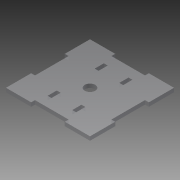
# Autodesk Inventor part: inside_box_top_bot
Saved by Autodesk Inventor 2013 (Build 170138000, 138)
## iProperties
Created: 2014-05-23
Part Number: inside_box_top_bot
Material: Polycarbonate, Clear
Document SubType Name: Modeling
Designer: balogh
Density: 0.894 g/cm^3
Mass: 9.34464 g
Surface Area: 83.2097 cm^2
Volume: 10.4526 cm^3
Author: balogh
Autodesk Inventor part; units mm, degrees
ref_plane "YZ Plane" through (0, 0, 0) normal (1, 0, 0) x (0, 1, 0)
ref_plane "XZ Plane" through (0, 0, 0) normal (0, 1, 0) x (-1, 0, 0)
ref_plane "XY Plane" through (0, 0, 0) normal (0, 0, 1) x (1, 0, 0)
sketch "Sketch1" plane through (0, 0, 0) normal (0, 0, 1) x (1, 0, 0)
  spline S0 degree 2 poles (0, 3.9053) (3.9053, 3.9053) (3.9053, 0) (3.9053, -3.9053) (0, -3.9052) (-3.9053, -3.9053) (-3.9052, 0) (-3.9052, 3.9053) (0, 3.9053) knots 0 0 0 0.24151 0.24151 0.48302 0.48302 0.72453 0.72453 0.96604 0.96604 0.96604 weights 1 0.707107 1 0.707107 1 0.707107 1 0.707107 1
  line L0 (0, 3.9053) -> (3.9053, 3.9053) construction
  line L1 (3.9053, 3.9053) -> (3.9053, 0) construction
  line L2 (3.9053, 0) -> (3.9053, -3.9053) construction
  line L3 (3.9053, -3.9053) -> (0, -3.9052) construction
  line L4 (0, -3.9052) -> (-3.9053, -3.9053) construction
  line L5 (-3.9053, -3.9053) -> (-3.9052, 0) construction
  line L6 (-3.9052, 0) -> (-3.9052, 3.9053) construction
  line L7 (-3.9052, 3.9053) -> (0, 3.9053) construction
  line L8 (-28.8544, 12.7) -> (-28.8544, -12.7)
  line L9 (-28.8544, -12.7) -> (-31.75, -12.7)
  line L10 (-31.75, -12.7) -> (-31.75, -31.75)
  line L11 (-31.75, -31.75) -> (-12.7, -31.75)
  line L12 (-12.7, -31.75) -> (-12.7, -28.8544)
  line L13 (-12.7, -28.8544) -> (12.7, -28.8544)
  line L14 (12.7, -28.8544) -> (12.7, -31.75)
  line L15 (12.7, -31.75) -> (31.75, -31.75)
  line L16 (31.75, -31.75) -> (31.75, -12.7)
  line L17 (31.75, -12.7) -> (28.8544, -12.7)
  line L18 (28.8544, -12.7) -> (28.8544, 12.7)
  line L19 (28.8544, 12.7) -> (31.75, 12.7)
  line L20 (31.75, 12.7) -> (31.75, 31.75)
  line L21 (31.75, 31.75) -> (12.7, 31.75)
  line L22 (12.7, 31.75) -> (12.7, 28.8544)
  line L23 (12.7, 28.8544) -> (-12.7, 28.8544)
  line L24 (-12.7, 28.8544) -> (-12.7, 31.75)
  line L25 (-12.7, 31.75) -> (-31.75, 31.75)
  line L26 (-31.75, 31.75) -> (-31.75, 12.7)
  line L27 (-31.75, 12.7) -> (-28.8544, 12.7)
  line L28 (21.2471, 10.7696) -> (14.3129, 10.7696)
  line L29 (14.3129, 10.7696) -> (14.3129, 7.874)
  line L30 (14.3129, 7.874) -> (21.2471, 7.874)
  line L31 (21.2471, 7.874) -> (21.2471, 10.7696)
  line L32 (-21.2471, 10.7696) -> (-14.3129, 10.7696)
  line L33 (-14.3129, 10.7696) -> (-14.3129, 7.874)
  line L34 (-14.3129, 7.874) -> (-21.2471, 7.874)
  line L35 (-21.2471, 7.874) -> (-21.2471, 10.7696)
  line L36 (-21.2471, -10.7696) -> (-14.3129, -10.7696)
  line L37 (-14.3129, -10.7696) -> (-14.3129, -7.874)
  line L38 (-14.3129, -7.874) -> (-21.2471, -7.874)
  line L39 (-21.2471, -7.874) -> (-21.2471, -10.7696)
  line L40 (21.2471, -10.7696) -> (14.3129, -10.7696)
  line L41 (14.3129, -10.7696) -> (14.3129, -7.874)
  line L42 (14.3129, -7.874) -> (21.2471, -7.874)
  line L43 (21.2471, -7.874) -> (21.2471, -10.7696)
  point P0 (0, 0)
  constraints: 72 end point, 23 parallel, 10 perpendicular, 2 collinear, 2 other
extrude "Extrusion1" add sketch "Sketch1" along normal blind 2.8956
body "Solid1"
